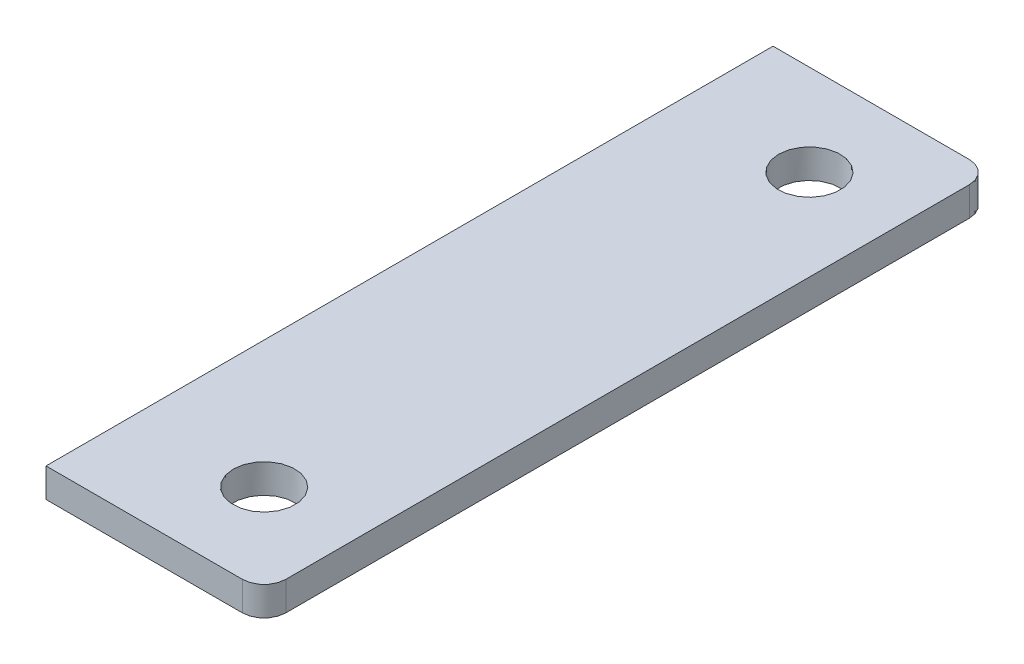
# Autodesk Inventor part: Ухо на швеллер пямое
Saved by Autodesk Inventor 2024.2 (Build 282272000, 272)
## iProperties
Created: 2024-06-15
Part Number: Ухо на швеллер пямое
Material: Generic
Document SubType Name: Sheet Metal
Designer: admin
Density: 1 g/cm^3
Sheet Metal Rule: Default
Appearance: Default
Author: admin
Autodesk Inventor part; units mm, degrees
ref_plane "YZ Plane" through (0, 0, 0) normal (1, 0, 0) x (0, 1, 0)
ref_plane "XZ Plane" through (0, 0, 0) normal (0, 1, 0) x (-1, 0, 0)
ref_plane "XY Plane" through (0, 0, 0) normal (0, 0, 1) x (1, 0, 0)
sketch "Sketch1" plane through (0, 0, 0) normal (0, 1, 0) x (-1, 0, 0)
  line L0 (0, 100) -> (-60, 100)
  line L1 (-60, 100) -> (-60, -100)
  line L2 (-60, -100) -> (0, -100)
  line L3 (0, -100) -> (0, 100)
  point P0 (0, 0)
  point P1 (0, 0)
  dimension "d0" = 60
  dimension "d1" = 200
  measures "d0" distance of L0.start L0.end
  measures "d1" distance of L2.end L0.start
extrude "Plate1" add sketch "Sketch1" along normal blind 8
sketch "Sketch2" plane through (0, 0, 0) normal (0, -1, 0) x (1, 0, 0)
  line L0 (35, 75) -> (35, -75) construction
  line L1 (0, -100) -> (0, 100) projected
  line L2 (60, 100) -> (60, -100) projected
  point P0 (0, 0)
  point P1 (35, 0)
  point P2 (0, 0)
  dimension "d10" = 25
  dimension "d12" = 25
  constraints: 2 end point, 2 midpoint, 1 coincident, 1 horizontal alignment, 1 vertical
  measures "d10" distance between parallel lines of L2 L0
  measures "d12" horizontal distance of L0.start L2.start
hole "Hole1" at (35, 0, 75) at (35, 0, -75) direction (0, 1, 0) diameter 17 end through all
fillet "Corner Round1" radius 6 2 edges at (60, 4, 100) (60, 4, -100)
equation "\"d12\" = d10"
equation "\"d8\" = Thickness"
equation "\"d2\" = Thickness"
equation "\"BendRadius\" = Thickness"
equation "\"BendReliefWidth\" = Thickness"
equation "\"BendReliefDepth\" = 0.5 * Thickness"
equation "\"CornerReliefSize\" = 4 * Thickness"
equation "\"MinimumRemnant\" = 2 * Thickness"
equation "\"TransitionRadius\" = BendRadius"
equation "\"JacobiRadiusSize\" = BendRadius"
equation "\"GapSize\" = Thickness"
equation "\"Thickness\" = 8"
body "Solid1"
